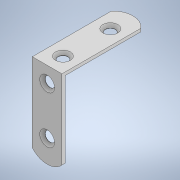
# Autodesk Inventor part: CornerBrace
Saved by Autodesk Inventor 2020 (Build 240168000, 168)
## iProperties
Created: 2021-11-11
Part Number: CornerBrace
Material: Generic
Document SubType Name: Modeling
Designer: 17185
Density: 1 g/cm^3
Appearance: Default
Author: 17185
Autodesk Inventor part; units mm, degrees
ref_plane "YZ Plane" through (0, 0, 0) normal (1, 0, 0) x (0, 1, 0)
ref_plane "XZ Plane" through (0, 0, 0) normal (0, 1, 0) x (-1, 0, 0)
ref_plane "XY Plane" through (0, 0, 0) normal (0, 0, 1) x (1, 0, 0)
sketch "Sketch4" plane through (0, 0, 0) normal (0, 1, 0) x (-1, 0, 0)
  line L0 (9.525, 25.4) -> (-9.525, 25.4)
  line L1 (-9.525, 25.4) -> (-9.525, -25.4)
  line L2 (-9.525, -25.4) -> (9.525, -25.4)
  line L3 (9.525, -25.4) -> (9.525, 25.4)
  line L4 (9.525, 25.4) -> (-9.525, -25.4) construction
  line L5 (-9.525, 25.4) -> (9.525, -25.4) construction
  arc A0 (-9.525, -25.4) -> (9.525, -25.4) centre (0, -16.9997) ccw
  point P0 (0, 0)
  dimension "d10" = 19.05
  dimension "d11" = 50.8
  dimension "d12" = 12.7
  constraints: 12 end point, 2 midpoint, 2 parallel, 2 point on circle, 1 centre point, 1 horizontal, 1 perpendicular
  measures "d10" distance of L2.end L1.end
  measures "d11" distance of L0.end L1.end
  measures "d12" radius of A0
extrude "Extrusion2" add sketch "Sketch4" along normal blind 1.9844
sketch "Sketch5" plane through (0, 1.9844, 0) normal (0, 1, 0) x (1, 0, 0)
  point P0 (0, 0)
  point P1 (0, 15.24)
  point P2 (0, -15.24)
  dimension "d15" = 15.24
  dimension "d16" = 15.24
  measures "d15" distance of point (0, 15.24) point (0, 0)
  measures "d16" distance of point (0, 0) point (0, -15.24)
hole "Hole1" at (0, 1.9844, -15.24) at (0, 1.9844, 15.24) direction (0, -1, 0) diameter 6.35 depth 15.6718 tip angle 118 countersink diameter 9.525 countersink angle 82
sketch "Sketch6" plane through (-9.525, 0, 25.4) normal (0, 0, 1) x (1, 0, 0)
  line L0 (0, 1.9844) -> (19.05, 1.9844)
  line L1 (19.05, 1.9844) -> (19.05, -48.8156)
  line L2 (19.05, -48.8156) -> (0, -48.8156)
  line L3 (0, -48.8156) -> (0, 1.9844)
  arc A0 (0, -48.8156) -> (19.05, -48.8156) centre (9.525, -40.4154) ccw
  point P0 (9.525, 0)
  dimension "d24" = 19.05
  dimension "d25" = 50.8
  dimension "d28" = 12.7
  constraints: 8 end point, 2 parallel, 2 point on circle, 1 centre point, 1 horizontal, 1 perpendicular
  measures "d24" distance of L1.end L2.end
  measures "d25" distance of L0.end L1.end
  measures "d28" radius of A0
extrude "Extrusion3" add sketch "Sketch6" against normal blind 1.9844
sketch "Sketch7" plane through (-9.525, 1.9844, 25.4) normal (0, 0, 1) x (1, 0, 0)
  line L0 (0, -50.8) -> (0, 0) construction
  line L1 (19.05, -1.9844) -> (19.05, -50.8) construction
  line L2 (0, 0) -> (19.05, 0) construction
  line L3 (19.05, 0) -> (19.05, -50.8) construction
  line L4 (19.05, -50.8) -> (0, -50.8) construction
  line L5 (0, -50.8) -> (0, 0) construction
  line L6 (9.525, -25.4) -> (19.05, -25.4) construction
  point P0 (9.525, -1.9844)
  point P1 (9.525, -10.16)
  point P2 (9.525, -40.64)
  dimension "d29" = 15.24
  dimension "d30" = 15.24
  constraints: 10 end point, 2 parallel, 1 horizontal, 1 midpoint, 1 perpendicular
  measures "d29" distance from line of point (9.525, -10.16) L6
  measures "d30" distance from line of point (9.525, -40.64) L6
hole "Hole2" at (0, -8.1756, 25.4) at (0, -38.6556, 25.4) direction (0, 0, -1) diameter 6.35 depth 15.6718 tip angle 118 countersink diameter 9.525 countersink angle 82
equation "\"d16\" = d15"
equation "\"d30\" = d29"
body "Solid2"
